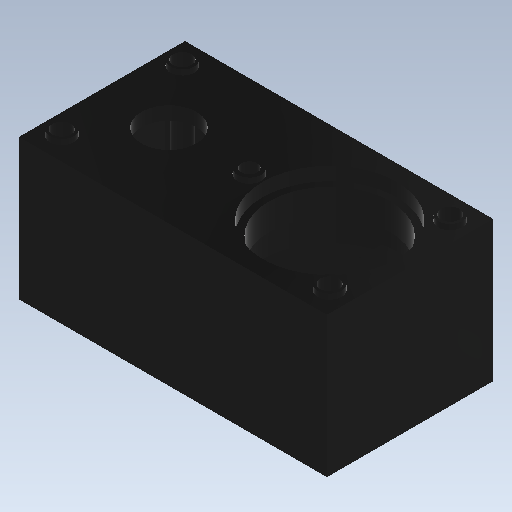
# Autodesk Inventor part: основание крпуса редуктора
Saved by Autodesk Inventor 2020 (Build 240168000, 168)
## iProperties
Created: 2018-08-24
Part Number: основание крпуса редуктора
Material: Пластик ПК/АБС
Document SubType Name: Modeling
Designer: Shepelev
Density: 0.357273 g/cm^3
Appearance: Гладкая - черная
Mass: 0.359508 g
Surface Area: 20.8611 cm^2
Volume: 1.00626 cm^3
Author: Shepelev
Autodesk Inventor part; units mm, degrees
ref_plane "YZ Plane" through (0, 0, 0) normal (1, 0, 0) x (0, 1, 0)
ref_plane "XZ Plane" through (0, 0, 0) normal (0, 1, 0) x (-1, 0, 0)
ref_plane "XY Plane" through (0, 0, 0) normal (0, 0, 1) x (1, 0, 0)
sketch "Эскиз1" plane through (0, 0, 0) normal (0, 1, 0) x (-1, 0, 0)
  line L0 (-11.5, 6.2) -> (11.5, 6.2)
  line L1 (11.5, 6.2) -> (11.5, -6.2)
  line L2 (11.5, -6.2) -> (-11.5, -6.2)
  line L3 (-11.5, -6.2) -> (-11.5, 6.2)
  line L4 (-11.5, 6.2) -> (11.5, -6.2) construction
  line L5 (11.5, 6.2) -> (-11.5, -6.2) construction
  point P0 (0, 0)
  dimension "d0" = 12.4
  dimension "d1" = 23
  constraints: 12 end point, 2 midpoint, 2 parallel, 1 horizontal, 1 perpendicular
  measures "d0" distance of L0.end L1.end
  measures "d1" distance of L1.end L2.end
extrude "Выдавливание1" add sketch "Эскиз1" along normal blind 10.5
sketch "Эскиз2" plane through (0, 0, 0) normal (0, -1, 0) x (1, 0, 0)
  line L0 (11.5, 6.2) -> (-11.5, 6.2) projected
  line L1 (-11.5, 6.2) -> (-11.5, -6.2) projected
  line L2 (-11.5, -6.2) -> (11.5, -6.2) projected
  line L3 (11.5, -6.2) -> (11.5, 6.2) projected
  line L4 (-10.5, 5.2) -> (10.5, 5.2)
  line L5 (10.5, 5.2) -> (10.5, -5.2)
  line L6 (10.5, -5.2) -> (-10.5, -5.2)
  line L7 (-10.5, -5.2) -> (-10.5, 5.2)
  point P0 (0, 0)
  dimension "d66" = 1
  constraints: 8 end point, 3 other
  measures "d66" distance between parallel lines of L2 L6
extrude "Выдавливание2" cut sketch "Эскиз2" against normal blind 9.5 contours L4 L5 L6 L7
chamfer "Фаска1" distance 1.5 angle 45 4 edges at (-10.5, 4.75, 5.2) (10.5, 4.75, 5.2) (10.5, 4.75, -5.2) (-10.5, 4.75, -5.2)
sketch "Эскиз3" plane through (0, 9.5, 0) normal (0, -1, 0) x (1, 0, 0)
  line L0 (9, -5.2) -> (-9, -5.2) projected
  line L1 (-4, -5.2) -> (-2.5, -3.7)
  line L2 (-2.5, -3.7) -> (-2.5, 3.7)
  line L3 (-2.5, 3.7) -> (-4, 5.2)
  line L4 (-9, 5.2) -> (9, 5.2) projected
  line L5 (-16.1, 0) -> (16.1, 0) projected
  line L6 (-10.5, -3.7) -> (-10.5, 3.7) projected
  line L7 (-2.5858, 5.2) -> (-1.5, 4.1142)
  line L8 (-1.5, 4.1142) -> (-1.5, -4.1142)
  line L9 (-1.5, -4.1142) -> (-2.5858, -5.2)
  point P0 (0, 0)
  dimension "d9" = 1.5
  dimension "d10" = 8
  dimension "d11" = 1
  dimension "d12" = 1
  constraints: 12 end point, 4 perpendicular, 4 point on line, 1 parallel, 1 other
  measures "d9" horizontal distance of L1.start L1.end
  measures "d10" distance between parallel lines of L2 L6
  measures "d11" distance between parallel lines of L8 L2
  measures "d12" distance between parallel lines of L7 L3
extrude "Выдавливание3" add sketch "Эскиз3" along normal blind 4
sketch "Эскиз4" plane through (0, 5.5, 0) normal (0, -1, 0) x (1, 0, 0)
  line L0 (-2.5, 3.7) -> (-2.5, -3.7) projected
  line L1 (-1.5, -4.1142) -> (-1.5, 4.1142) projected
  line L2 (-2.5, 3.7) -> (-1.5, 3.7)
  line L3 (-1.5, 3.7) -> (-1.5, -3.7)
  line L4 (-1.5, -3.7) -> (-2.5, -3.7)
  line L5 (-2.5, -3.7) -> (-2.5, 3.7)
  point P0 (0, 0)
  constraints: 8 end point, 2 parallel, 1 horizontal, 1 perpendicular, 1 point on line
extrude "Выдавливание4" add sketch "Эскиз4" along normal blind 1
sketch "Эскиз5" plane through (0, 9.5, 0) normal (0, -1, 0) x (1, 0, 0)
  line L0 (-10.5, -3.7) -> (-10.5, 3.7) projected
  line L1 (-2.5, -3.7) -> (-2.5, 3.7) projected
  line L2 (-9, 5.2) -> (9, 5.2) projected
  line L3 (9, -5.2) -> (-9, -5.2) projected
  line L4 (-2.5, 3.7) -> (-2.5, -3.7) projected
  point P0 (0, 0)
  point P1 (-6.5, 0)
  point P2 (-2.5, 0)
  dimension "d64" = 8
  dimension "d65" = 4
  constraints: 1 horizontal alignment, 1 midpoint
  measures "d64" distance between parallel lines of L0 L1
  measures "d65" distance from line of point (-6.5, 0) L1
hole "Отверстие1" at (-6.5, 9.5, 0) direction (0, 1, 0) diameter 4.1 depth 8 tip angle 118
sketch "Эскиз6" plane through (0, 9.5, 0) normal (0, -1, 0) x (1, 0, 0)
  circle A0 centre (5.5, 0) radius 5
  line L0 (10.5, 3.7) -> (10.5, -3.7) projected
  line L1 (-16.1, 0) -> (16.1, 0) projected
  line L2 (10.5, 3.7) -> (10.5, -3.7) projected
  circle A1 centre (5.5, 0) radius 6
  point P0 (0, 0)
  dimension "d24" = 10
  dimension "d25" = 1
  constraints: 2 centre point, 1 point on line, 1 tangent
  measures "d24" diameter of A0
  measures "d25" radial gap between concentric circles of A0 A1
extrude "Выдавливание5" add sketch "Эскиз6" along normal blind 4 contours L0 A1 L1 A0 | A0 L1 A1 L0 | L1 A1 L0 | L0 A1 L1
sketch "Эскиз7" plane through (5.5, 9.5, 0) normal (0, -1, 0) x (1, 0, 0)
  circle A0 centre (0, 0) radius 5 projected
  circle A1 centre (0, 0) radius 4.5
  point P0 (-5.5, 0)
  dimension "d28" = 9
  constraints: 1 centre point
  measures "d28" diameter of A1
extrude "Выдавливание6" cut sketch "Эскиз7" against normal blind 5 contours A1
sketch "Эскиз8" plane through (5.5, 9.5, 0) normal (0, -1, 0) x (1, 0, 0)
  circle A0 centre (0, 0) radius 4.5 projected
  circle A1 centre (0, 0) radius 5 projected
  point P0 (-5.5, 0)
extrude "Выдавливание7" add sketch "Эскиз8" along normal blind 2
sketch "Эскиз9" plane through (0, 10.5, 0) normal (0, 1, 0) x (1, 0, 0)
  circle A0 centre (5.5, 0) radius 4.5 projected
  circle A1 centre (5.5, 0) radius 5
  point P0 (0, 0)
  dimension "d33" = 10
  constraints: 1 centre point
  measures "d33" diameter of A1
extrude "Выдавливание8" cut sketch "Эскиз9" against normal blind 1
sketch "Эскиз10" plane through (0, 5.5, 0) normal (0, -1, 0) x (1, 0, 0)
  line L0 (2.5067, 5.2) -> (8.4933, 5.2) projected
  line L1 (4.5, 5.2) -> (6.5, 5.2)
  line L2 (6.5, 5.2) -> (6.5, 3.2)
  line L3 (6.5, 3.2) -> (4.5, 3.2)
  line L4 (4.5, 3.2) -> (4.5, 5.2)
  line L5 (9, -5.2) -> (-9, -5.2) projected
  line L6 (4.5, -5.2) -> (6.5, -5.2)
  line L7 (6.5, -5.2) -> (6.5, -3.2)
  line L8 (6.5, -3.2) -> (4.5, -3.2)
  line L9 (4.5, -3.2) -> (4.5, -5.2)
  line L10 (-16.1, 0) -> (16.1, 0) projected
  circle A0 centre (5.5, 0) radius 4.5 projected
  point P0 (0, 0)
  point P1 (5.5, 3.2)
  dimension "d36" = 2
  dimension "d37" = 2
  constraints: 16 end point, 4 parallel, 2 horizontal, 2 perpendicular, 2 point on line, 1 midpoint, 1 vertical alignment, 3 other
  measures "d36" distance of L1.end L2.end
  measures "d37" distance of L2.end L3.end
extrude "Выдавливание9" add sketch "Эскиз10" against normal blind 0.5 contours L0 L2 A0 L4 | A0 L2 L3 L4 | A0 L7 L5 L9 | L9 L8 L7 A0
sketch "Эскиз11" plane through (0, 9.5, 0) normal (0, -1, 0) x (1, 0, 0)
  circle A0 centre (-0.5, 0) radius 1
  line L0 (-11.5, 6.2) -> (-11.5, -6.2) projected
  point P0 (0, 0)
  dimension "d40" = 11
  dimension "d41" = 2
  constraints: 1 centre point
  measures "d40" distance from line of L0 A0.centre
  measures "d41" diameter of A0
extrude "Выдавливание10" add sketch "Эскиз11" along normal blind 2
sketch "Эскиз12" plane through (0, 10.5, 0) normal (0, 1, 0) x (1, 0, 0)
  arc A0 (-1.5, 0) -> (-0.4167, -0.9965) centre (-0.5, 0) ccw projected
  line L0 (-11.5, 6.2) -> (-11.5, -6.2) projected
  circle A1 centre (-6.428, 0) radius 2.05 projected
  point P0 (0, 0)
  point P1 (-1.5, -0.866)
  dimension "d63" = 11
  constraints: 1 other
  measures "d63" distance from line of L0 point (-0.5, 0)
hole "Отверстие2" at (-0.5, 10.5, 0) direction (0, -1, 0) diameter 1.2 depth 2
sketch "Эскиз13" plane through (0, 0, 0) normal (0, -1, 0) x (1, 0, 0)
  line L0 (-10, -4.5) -> (10, -4.5)
  line L1 (10, -4.5) -> (10, 4.5)
  line L2 (10, 4.5) -> (-10, 4.5)
  line L3 (-10, 4.5) -> (-10, -4.5)
  line L4 (-10, -4.5) -> (10, 4.5) construction
  line L5 (10, -4.5) -> (-10, 4.5) construction
  point P0 (0, 0)
  dimension "d51" = 9
  dimension "d52" = 20
  constraints: 12 end point, 2 midpoint, 2 parallel, 1 horizontal, 1 perpendicular
  measures "d51" distance of L0.end L1.end
  measures "d52" distance of L1.end L2.end
hole "Отверстие3" at (10, 0, 4.5) at (10, 0, -4.5) at (-10, 0, 4.5) at (-10, 0, -4.5) direction (0, 1, 0) diameter 1.4 depth 12 tip angle 118
sketch "Эскиз14" plane through (0, 10.5, 0) normal (0, 1, 0) x (1, 0, 0)
  circle A0 centre (10, 4.5) radius 0.7 projected
  circle A1 centre (10, -4.5) radius 0.7 projected
  circle A2 centre (-10, -4.5) radius 0.7 projected
  circle A3 centre (-10, 4.5) radius 0.7 projected
  circle A4 centre (10, 4.5) radius 0.9
  circle A5 centre (-10, 4.5) radius 0.9
  circle A6 centre (-10, -4.5) radius 0.9
  circle A7 centre (10, -4.5) radius 0.9
  circle A8 centre (-0.5, 0) radius 0.6 projected
  circle A9 centre (-0.5, 0) radius 0.9
  point P0 (0, 0)
  dimension "d60" = 1.8
  constraints: 5 centre point, 4 equal radius
  measures "d60" diameter of A4
extrude "Выдавливание11" add sketch "Эскиз14" along normal blind 0.4
equation "\"d65\" = 0.5 * d64"
